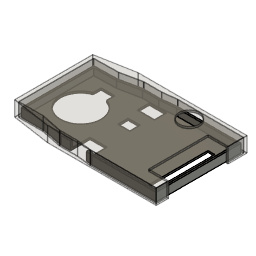
Case-Electronics (Autodesk Fusion 360 design; units mm, degrees)
Autodesk Fusion 360 part; units mm, degrees
sketch "Sketch1" plane through (0, 0, 0) normal (0, 1, 0) x (1, 0, 0)
  line L0 (0, 0) -> (18, 0)
  line L1 (18, 0) -> (18, 45)
  line L2 (18, 45) -> (0, 45)
  line L3 (0, 45) -> (0, 0)
  line L4 (19.0267, -1) -> (54.0267, -1)
  line L5 (54.0267, -1) -> (54.0267, 46)
  line L6 (54.0267, 46) -> (19.0267, 46)
  line L7 (19.0267, 46) -> (19.0267, -1)
  line L8 (54.5267, 46.5) -> (18.5267, 46.5)
  line L9 (18.5267, 46.5) -> (18.5267, -1.5)
  line L10 (18.5267, -1.5) -> (54.5267, -1.5)
  line L11 (54.5267, -1.5) -> (54.5267, 46.5)
  line L12 (55.5267, 47.5) -> (17.5267, 47.5)
  line L13 (17.5267, 47.5) -> (17.5267, -2.5)
  line L14 (17.5267, -2.5) -> (55.5267, -2.5)
  line L15 (55.5267, -2.5) -> (55.5267, 47.5)
  line L16 (18.5, 45.5) -> (-0.5, 45.5)
  line L17 (-0.5, 45.5) -> (-0.5, -0.5)
  line L18 (-0.5, -0.5) -> (18.5, -0.5)
  line L19 (18.5, -0.5) -> (18.5, 45.5)
  line L20 (19.5, 46.5) -> (-1.5, 46.5)
  line L21 (-1.5, 46.5) -> (-1.5, -1.5)
  line L22 (-1.5, -1.5) -> (19.5, -1.5)
  line L23 (19.5, -1.5) -> (19.5, 46.5)
  line L24 (17.5267, -2.5) -> (9, -1.5)
  line L25 (17.5267, 47.5) -> (9, 46.5)
  line L26 (9, 45.5) -> (18.5267, 46.5)
  line L27 (9, 0) -> (18.5267, -1.5)
  line L28 (49.532, 38.0472) -> (45.532, 38.0472)
  line L29 (45.532, 38.0472) -> (45.532, 3.0472)
  line L30 (45.532, 3.0472) -> (49.532, 3.0472)
  line L31 (49.532, 3.0472) -> (49.532, 38.0472)
  line L32 (9, 0) -> (14, 0)
  line L33 (9, 0) -> (4, 0)
  line L34 (4, 0) -> (14, 0)
  line L35 (14, 0) -> (14, 10)
  line L36 (14, 10) -> (4, 10)
  line L37 (4, 10) -> (4, 0)
  line L38 (4, 0) -> (4, -1.5)
  line L39 (14, 0) -> (14, -2.0864)
  line L40 (9, 45) -> (4, 45)
  line L41 (9, 45) -> (14, 45)
  line L42 (14, 45) -> (14, 38)
  line L43 (14, 38) -> (4, 38)
  line L44 (4, 38) -> (4, 45)
  line L45 (9, 45) -> (9, 25)
  line L46 (9, 25) -> (5.5, 25)
  line L47 (5.5, 25) -> (12.5, 25)
  line L48 (12.5, 25) -> (12.5, 31)
  line L49 (12.5, 31) -> (5.5, 31)
  line L50 (5.5, 31) -> (5.5, 25)
  line L51 (0, 22.5) -> (-26, 22.5)
  line L52 (-26, 22.5) -> (-26, 42.17)
  line L53 (-26, 22.5) -> (-26, 2.512)
  line L54 (-26, 42.17) -> (0, 42.6767)
  line L55 (-26, 2.512) -> (0, 2.5357)
  line L56 (-26.5, 22.5) -> (-26.5, 42.6603)
  line L57 (-26.5, 42.6603) -> (0, 43.1768)
  line L58 (-26.5, 22.5) -> (-26.5, 2.0115)
  line L59 (-26.5, 2.0115) -> (0, 2.0357)
  line L60 (-27.5, 22.6912) -> (-27.5, 1.0106)
  line L61 (-27.5, 1.0106) -> (0, 1.0357)
  line L62 (-27.5, 22.6912) -> (-27.5, 43.641)
  line L63 (-27.5, 43.641) -> (0, 44.177)
  line L64 (-13.25, 42.9185) -> (-0.5, 45.5)
  line L65 (-13.75, 43.909) -> (-1.5, 46.5)
  line L66 (-13.75, 1.0232) -> (-1.5, -1.5)
  line L67 (-13.25, 2.0236) -> (-0.5, -0.5)
  line L68 (-26, 42.17) -> (-26, 2.512)
  circle A0 centre (-14, 22.5) radius 12
  line L69 (-14, 34.5) -> (-18, 34.5)
  line L70 (-18, 34.5) -> (-10, 34.5)
  line L71 (-18, 34.5) -> (-18, 38.5)
  line L72 (-18, 38.5) -> (-10, 38.5)
  line L73 (-10, 38.5) -> (-10, 34.5)
  line L74 (-18, 34.5) -> (-18, 33.8137)
  line L75 (-10, 34.5) -> (-10, 33.8137)
  line L76 (17.5267, -3.3) -> (56.3267, -3.3)
  line L77 (56.3267, -3.3) -> (56.3267, 48.3)
  line L78 (56.3267, 48.3) -> (17.5267, 48.3)
  line L79 (17.4335, 48.2946) -> (8.9532, 47.3)
  line L80 (19.5, 47.3) -> (-1.5, 47.3)
  line L81 (-28.3, 44.4256) -> (-0.0095, 44.9769)
  line L82 (-28.3, 22.6912) -> (-28.3, 44.4256)
  line L83 (-28.3, 22.6912) -> (-28.3, 0.2099)
  line L84 (-28.3, 0.2099) -> (0.0007, 0.2357)
  line L85 (-13.9114, 0.2396) -> (-1.6614, -2.2836)
  line L86 (-1.5, -2.3) -> (20.3, -2.3)
  line L87 (20.3, -2.3) -> (20.3, 47.3)
  line L88 (20.3, 47.3) -> (-1.5, 47.3)
  line L89 (-1.6614, -2.2836) -> (-1.5, -2.3)
  line L90 (17.4335, -3.2946) -> (8.9532, -2.3)
  line L91 (17.4335, -3.2946) -> (17.5267, -3.3)
  line L92 (17.4335, 48.2946) -> (17.5267, 48.3)
  line L93 (-1.6654, 47.2827) -> (-1.5, 47.3)
  line L94 (-13.8414, 44.7074) -> (-1.6654, 47.2827)
  line L95 (56.3267, 48.3) -> (57.3873, 49.3607)
  line L96 (56.3267, 48.3) -> (57.8267, 48.3) construction
  line L97 (57.3873, 49.3607) -> (-29.6127, 49.3607)
  line L98 (-29.6127, 49.3607) -> (-29.6127, -4.3393)
  line L99 (-29.6127, -4.3393) -> (57.3873, -4.3393)
  line L100 (57.3873, -4.3393) -> (57.3873, 49.3607)
  line L101 (-29.6127, 45.2022) -> (-6.9658, 49.3607)
  line L102 (-29.6127, -0.9415) -> (-6.7269, -4.3393)
  line L103 (49.532, 3.0472) -> (57.3873, 3.0472)
  line L104 (49.532, 38.0472) -> (57.3873, 38.0472)
  line L105 (47.532, 38.0472) -> (31.532, 38.0472)
  line L106 (31.532, 46) -> (31.532, 41)
  circle A1 centre (31.532, 41) radius 6
  dimension "d1" = 18
  dimension "d2" = 45
  dimension "d3" = 35
  dimension "d4" = 47
  dimension "d5" = 0.5
  dimension "d6" = 1.5
  dimension "d7" = 0.5
  dimension "d8" = 1.5
  dimension "d13" = 4
  dimension "d14" = 35
  dimension "d15" = 5
  dimension "d16" = 5
  dimension "d17" = 10
  dimension "d18" = 10
  dimension "d19" = 5
  dimension "d20" = 5
  dimension "d21" = 7
  dimension "d22" = 20
  dimension "d24" = 3.5
  dimension "d25" = 7
  dimension "d26" = 6
  dimension "d27" = 26
  dimension "d30" = -0.5
  dimension "d31" = 0.5
  dimension "d32" = 1.5
  dimension "d33" = -1.5
  dimension "d34" = 24
  dimension "d38" = 4
  dimension "d39" = 8
  dimension "d40" = 4
  dimension "d41" = 8
  dimension "d42" = 0.8
  dimension "d43" = 0.8
  dimension "d44" = 0.8
  dimension "d46" = -0.8
  dimension "d47" = 0.8
  dimension "d48" = 0.8
  dimension "d49" = -0.8
  dimension "d50" = 45
  dimension "d51" = 1.5
  dimension "d52" = 87
  dimension "d53" = 53.7
  dimension "d59" = 16
  dimension "d60" = 5
  dimension "d61" = 12
  constraint horizontal L0
  constraint vertical L1
  constraint horizontal L2
  constraint vertical L3
  constraint coincident L0.start L3.end
  constraint horizontal L4
  constraint vertical L5
  constraint horizontal L6
  constraint vertical L7
  constraint midpoint L22 L24.end
  constraint midpoint L20 L25.end
  constraint midpoint L16 L26.start
  constraint midpoint L0 L27.start
  constraint horizontal L28
  constraint vertical L29
  constraint horizontal L30
  constraint vertical L31
  constraint parallel L0 L32
  constraint parallel L0 L33
  constraint horizontal L34
  constraint vertical L35
  constraint horizontal L36
  constraint vertical L37
  constraint coincident L22 L38.end
  constraint perpendicular L22 L38
  constraint coincident L24 L39.end
  constraint perpendicular L22 L39
  constraint midpoint L2 L40.start
  constraint coincident L2 L40.end
  constraint parallel L2 L41
  constraint perpendicular L2 L42
  constraint perpendicular L42 L43
  constraint perpendicular L40 L44
  constraint perpendicular L43 L45
  constraint perpendicular L45 L46
  constraint horizontal L47
  constraint vertical L48
  constraint horizontal L49
  constraint vertical L50
  constraint midpoint L3 L51.start
  constraint perpendicular L17 L51
  constraint perpendicular L51 L52
  constraint perpendicular L51 L53
  constraint coincident L3 L54.end
  constraint coincident L3 L55.end
  constraint coincident L3 L59.end
  constraint coincident L3 L57.end
  constraint coincident L3 L63.end
  constraint coincident L3 L61.end
  constraint midpoint L57 L64.start
  constraint midpoint L63 L65.start
  constraint midpoint L61 L66.start
  constraint midpoint L59 L67.start
  constraint coincident A0 L69.start
  constraint tangent A0 L69
  constraint parallel L51 L69
  constraint parallel L69 L70
  constraint perpendicular L69 L71
  constraint perpendicular L62 L72
  constraint coincident A0 L74.end
  constraint perpendicular L69 L74
  constraint coincident A0 L75.end
  constraint perpendicular L70 L75
  constraint coincident L86 L90.end
  constraint coincident L79.end L88
  constraint coincident L81 L94.start
  constraint horizontal L96
  constraint horizontal L97
  constraint vertical L98
  constraint horizontal L99
  constraint vertical L100
  constraint coincident L98 L101.start
  constraint coincident L97 L101.end
  constraint coincident L98 L102.start
  constraint coincident L99 L102.end
  constraint coincident L100 L103.end
  constraint perpendicular L100 L103
  constraint coincident L100 L104.end
  constraint perpendicular L100 L104
  constraint midpoint L28 L105.start
  constraint perpendicular L29 L105
  constraint coincident L6 L106.start
  constraint perpendicular L6 L106
  constraint coincident L106.end A1.centre
  measures "d1" distance of L0.start L0.end
  measures "d2" distance of L0.start L2.end
  measures "d3" distance of L4.start L4.end
  measures "d4" distance of L4.start L6.end
  measures "d13" distance of L28.start L28.end
  measures "d14" distance of L28.start L30.end
  measures "d15" distance of L27.start L32.end
  measures "d16" distance of L27.start L33.end
  measures "d17" distance of L33.end L32.end
  measures "d18" distance of L33.end L36.end
  measures "d19" distance of L40.start L40.end
  measures "d20" distance of L40.start L41.end
  measures "d21" distance of L41.end L42.end
  measures "d22" distance of L40.start L45.end
  measures "d24" distance of L45.end L46.end
  measures "d25" distance of L46.end L47.end
  measures "d26" distance of L46.end L49.end
  measures "d27" distance of L51.start L51.end
  measures "d34" diameter of A0
  measures "d38" distance of L69.start L69.end
  measures "d39" distance of L69.end L70.end
  measures "d40" distance of L69.end L71.end
  measures "d41" distance of L71.end L72.end
  measures "d50" angle of L95 L96
  measures "d51" distance of L77.end L95.end
  measures "d52" distance of L95.end L97.end
  measures "d53" distance of L95.end L99.end
  measures "d59" distance of L105.start L105.end
  measures "d60" distance of L106.start L106.end
  measures "d61" diameter of A1
extrude "Extrude1" add sketch "Sketch1" along normal blind 5 contours L18 L21 L22 L38 L67 | L13 L22 L27 L39 | L21 L66 L67 L84 | L61 L66 L67 L84 | L13 L22 L27 | L13 L22 L24 L39 L86 | L56 L57 L58 L59 L60 L61 L62 L63 L64 L67 | L10 L13 L22 L86 L87 | L13 L24 L86 | L13 L16 L20 L21 L26 L64 | L13 L20 L26 | L10 L11 L13 L14 L15 L86 L87 L103 | L8 L13 L20 L80 L87 L88 | L13 L20 L25 L80 L88 | L13 L25 L80 L88 | L8 L11 L12 L13 L15 L80 L87 L88 L104 A1 | L21 L64 L65 L81 | L11 L15 L103 L104 | L63 L64 L65 L81 | L8 A1 makes body 1
extrude "Extrude2" add sketch "Sketch1" 1 faces at (-4.8313, 0, -45.4003) along normal blind 1 contours L0 L2 L3 L13 L35 L36 L37 L42 L43 L44 | L0 L3 L17 L18 L38 L84 | L3 L17 L61 L84 | L18 L21 L22 L38 L67 | L3 L17 L59 L61 | L17 L21 L61 L84 | L17 L21 L67 L84 | L0 L13 L18 L39 | L3 L17 L55 L59 | L17 L21 L59 L61 | L21 L61 L67 L84 | L21 L67 L84 | L0 L1 L2 L13 | L0 L1 L2 L13 L16 L18 L19 | L13 L18 L27 L39 | L13 L22 L27 L39 | L3 L17 L51 L55 | L17 L21 L55 L59 | L21 L59 L61 L67 | L2 L3 L13 L16 L17 L40 L41 L63 | L9 L13 L16 L18 L19 L26 L27 | L13 L22 L27 | L13 L22 L24 L39 L86 | L3 L17 L51 L54 | L17 L21 L51 L55 | L21 L52 L53 L54 L55 L56 L57 L58 L59 L68 | L13 L16 L26 | L10 L13 L22 L86 L87 | L4 L6 L7 L8 L9 L10 L20 L22 L23 | L13 L24 L86 | L3 L17 L54 L57 | L17 L21 L51 L54 | L21 L51 L53 L55 L68 A0 | L13 L16 L20 L21 L26 L64 | L13 L20 L26 | L10 L11 L13 L14 L15 L86 L87 L103 | L8 L13 L20 L80 L87 L88 | L4 L10 L23 L87 | L3 L17 L57 L63 | L17 L21 L54 L57 | L21 L51 L52 L54 L68 A0 L71 L72 L73 L74 L75 | L13 L20 L25 L80 L88 | L17 L21 L64 L81 | L6 L8 L23 L87 | L4 L5 L10 L11 L87 L103 | L4 L6 L23 L87 | L4 L6 L7 L23 | L17 L21 L57 L63 | L13 L25 L80 L88 | L8 L11 L12 L13 L15 L80 L87 L88 L104 A1 | L17 L21 L63 L81 | L21 L64 L81 | L6 L8 L87 A1 | L4 L5 L6 L29 L30 L87 L103 L105 A1 | L11 L15 L103 L104 | L21 L57 L63 L64 | L21 L63 L64 L81 | L8 A1 | L6 L8 A1 | L5 L11 L103 L104 | L5 L6 L8 L11 L104 A1 | L6 A1 | L5 L31 L103 L104 | L5 L6 L28 L104 L105 A1 on bodies 1 bodies 1
extrude "Extrude3" add sketch "Sketch1" along normal blind 9 separate body contours L76 L77 L78 L79 L80 L81 L82 L83 L84 L85 L86 L88 L89 L90 L91 L92 L93 L94 L95 L97 L98 L99 L100 L101 L102 L103 | L77 L95 L100 L104 makes body 2
extrude "Extrude5" add sketch "Sketch1" along normal blind 1 from surface at 8 contours L0 L2 L3 L13 L35 L36 L37 L42 L43 L44 | L0 L3 L17 L18 L38 L84 | L0 L32 L33 L34 L35 L36 L37 | L0 L18 L27 L33 L34 L38 | L3 L17 L61 L84 | L0 L18 L27 L32 L34 L39 | L18 L21 L22 L38 L67 | L18 L22 L27 L38 L39 | L3 L17 L59 L61 | L17 L21 L61 L84 | L17 L21 L67 L84 | L0 L13 L18 L39 | L18 L27 L39 | L22 L24 L66 L84 L85 L86 L89 | L3 L17 L55 L59 | L17 L21 L59 L61 | L21 L61 L67 L84 | L21 L67 L84 | L0 L1 L2 L13 | L0 L1 L2 L13 L16 L18 L19 | L13 L18 L27 L39 | L13 L22 L27 L39 | L21 L66 L67 L84 | L22 L24 L39 | L3 L17 L51 L55 | L17 L21 L55 L59 | L21 L59 L61 L67 | L61 L66 L67 L84 | L2 L3 L13 L16 L17 L40 L41 L63 | L9 L13 L16 L18 L19 L26 L27 | L13 L22 L27 | L13 L22 L24 L39 L86 | L60 L61 L62 L63 L65 L66 L81 L82 L83 L84 | L3 L17 L51 L54 | L17 L21 L51 L55 | L21 L52 L53 L54 L55 L56 L57 L58 L59 L68 | L56 L57 L58 L59 L60 L61 L62 L63 L64 L67 | L2 L41 L42 L43 L45 | L13 L16 L26 | L10 L13 L22 L86 L87 | L4 L6 L7 L8 L9 L10 L20 L22 L23 | L13 L24 L86 | L14 L15 L24 L76 L77 L86 L90 L91 L103 | L3 L17 L54 L57 | L17 L21 L51 L54 | L21 L51 L53 L55 L68 A0 | L2 L40 L43 L44 L45 | L13 L16 L20 L21 L26 L64 | L13 L20 L26 | L10 L11 L13 L14 L15 L86 L87 L103 | L8 L13 L20 L80 L87 L88 | L4 L10 L23 L87 | L3 L17 L57 L63 | L17 L21 L54 L57 | L21 L51 L52 L54 L68 A0 L71 L72 L73 L74 L75 | L13 L20 L25 L80 L88 | L17 L21 L64 L81 | L6 L8 L23 L87 | L4 L5 L10 L11 L87 L103 | L4 L6 L23 L87 | L4 L6 L7 L23 | L17 L21 L57 L63 | L51 A0 | L51 A0 | L13 L25 L80 L88 | L8 L11 L12 L13 L15 L80 L87 L88 L104 A1 | L20 L25 L65 L80 L81 L88 L93 L94 | L17 L21 L63 L81 | L21 L64 L65 L81 | L21 L64 L81 | L6 L8 L87 A1 | L4 L5 L6 L29 L30 L87 L103 L105 A1 | L21 L57 L63 L64 | A0 L70 L75 | A0 L69 L70 L74 | L12 L15 L25 L77 L78 L79 L80 L88 L92 L104 | L21 L63 L64 L81 | L63 L64 L65 L81 | L69 L70 L71 L72 L73 | L5 L6 L8 L11 L104 A1 | L5 L6 L28 L104 L105 A1 | L45 L47 L48 L49 | L45 L46 L47 L49 L50 bodies 2
